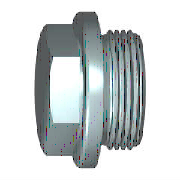
# Autodesk Inventor part: CSN 02 1915.21 - M 20 x 10
Saved by Autodesk Inventor 2016 (Build 200138000, 138)
## iProperties
Created: 2015-02-19
Part Number: CSN 02 1915.21 - M 20 x 10
Material: Сталь, мягкая
Description: Пробка резьбовая с цилиндрической резьбой
Document SubType Name: Modeling
Standard: CSN 02 1915.21
Designer: Лол
Standards Organization: CSN
Language: ru-RU
Size Designation: M 20 x 10
Categories: <MemberInstance><Categories><Category DisplayName="Другие детали" InternalName="5aa15e00-363f-49f2-933f-16f664388e3f" Mnemonic="OTHER"><Category DisplayName="Пробки" InternalName="cac7eb15-d262-4465-a909-3aa76acf7ccc" Mnemonic="PGCLOS"><CategoryParameter DisplayName="Номинальный диаметр" InternalName="0cc7991d-0c39-4ac8-8486-c7d2ae5a3476" Mnemonic="nomdia2"/><CategoryParameter DisplayName="Обозначение серии резьб" InternalName="103883d0-9ece-47bf-a0f3-82d73a20391a" Mnemonic="thrserdsgn2"/><CategoryParameter DisplayName="Шаг резьбы" InternalName="3d473a7f-1ce0-4f16-9b77-af7fe5847f9b" Mnemonic="pitch2"/><CategoryParameter DisplayName="Витков на единицу" InternalName="705c2615-1a74-4f7a-b097-68f368d5139c" Mnemonic="thrperunit2"/><CategoryParameter DisplayName="Класс резьбы" InternalName="af44356c-65bc-4d9d-8b82-abec66cec71c" Mnemonic="thrclss2"/><CategoryParameter DisplayName="Обозначение резьбы" InternalName="d850c9d1-8a6b-401c-92c1-7eca3a245b93" Mnemonic="thrdesign2"/></Category></Category><Category DisplayName="ТипДанных" InternalName="23b78d0f-2648-40c6-8793-ca6db495c9e8" Mnemonic="DATATYPE"><CategoryParameter DisplayName="ОтображаемоеИмя" InternalName="05415f3d-3907-474b-a020-eb9d644f4cf3" Mnemonic="DISPLAYNAME"/><CategoryParameter DisplayName="Стандарт" InternalName="0c0a119c-1e12-4c84-803f-101930972f5e" Mnemonic="STANDARD"/><CategoryParameter DisplayName="Наименование" InternalName="13903e3d-64b1-4950-80da-f627842ea37f" Mnemonic="DESCRIPTION"/><CategoryParameter DisplayName="Обозначение" InternalName="2675968c-4ce5-49e0-a4f5-552d29089031" Mnemonic="DESIGNATION"/><CategoryParameter DisplayName="Строка по умолчанию" InternalName="2af9ec52-faaa-4026-b378-f9fa4afca842" Mnemonic="DEFAULTROW"/><CategoryParameter DisplayName="Имя папки" InternalName="3f06958e-8713-4116-9be7-ed6184ecc97b" Mnemonic="FOLDERNAME"/><CategoryParameter DisplayName="Указатель редакций" InternalName="45a75005-10b1-4dfc-8d6d-dfe629f0b93c" Mnemonic="REVISIONGUID"/><CategoryParameter DisplayName="ИмяФайла" InternalName="8b46a4cc-9585-4fed-90c3-899f57e09a73" Mnemonic="FILENAME"/><CategoryParameter DisplayName="ОргСтанд" InternalName="8f5914e1-4693-403f-8ab5-d37768198c9d" Mnemonic="STDSORG"/><CategoryParameter DisplayName="Версия семейства" InternalName="914462f6-6e19-4b14-ba84-155b9680b1d0" Mnemonic="FAMILYREVISION"/><CategoryParameter DisplayName="Редакция стандарта" InternalName="91d5a463-65c2-4fde-b823-3b7fea5e8e17" Mnemonic="STANDARDREVISION"/><CategoryParameter DisplayName="редакция элемента" InternalName="a65d44b9-392f-4f4f-857b-e4b3d54996fe" Mnemonic="MEMBERREVISION"/><CategoryParameter DisplayName="ФорматКлипа" InternalName="bc51e27b-3422-4e78-93ef-cec197ddf230" Mnemonic="CLIPFORMAT"/><CategoryParameter DisplayName="Изготовитель" InternalName="cd6c7a72-a28a-4e50-99a9-2c7f4e13e5ad" Mnemonic="MANUFACTURER"/><CategoryParameter DisplayName="ВнутреннееИмя" InternalName="cf1d0246-76d9-4b4a-8305-fa0409afb5c1" Mnemonic="INTERNALNAME"/><CategoryParameter DisplayName="Метрическая" InternalName="e2385c5b-1ea4-4823-96a8-8de651266ec3" Mnemonic="ISMETRIC"/><Category DisplayName="Деталь" InternalName="c0e0b642-3bcb-4cc8-9e80-f96d35c4afa4" Mnemonic="PART"><CategoryParameter DisplayName="Номер детали" InternalName="016b6077-bfbe-49bd-92c9-d8d59c39c941" Mnemonic="PARTNUMBER"/><CategoryParameter DisplayName="Инвентарный номер" InternalName="4dba7c1c-e26c-444e-836c-b08b433409a8" Mnemonic="STOCKNUMBER"/><CategoryParameter DisplayName="Ключ материала" InternalName="5c9a8adb-dd2b-4535-b97f-0a94a95fe41f" Mnemonic="MATERIALKEY"/><CategoryParameter DisplayName="Материал" InternalName="818a152a-d3c3-49ca-80ee-df7d91421b8e" Mnemonic="MATERIAL"/></Category></Category><Category DisplayName="СтараяКарта" InternalName="cd87c42b-3e48-431e-b5c0-1cbeb14dfe77" Mnemonic="LEGACYMAP"><CategoryParameter DisplayName="уникальное обозначение элемента DA" InternalName="0918ad47-427f-4fed-ae26-24c81c58f590" Mnemonic="DACOOKIE"/><CategoryParameter DisplayName="Объединить код 11" InternalName="0ee8fb18-e2ed-4f39-96f6-1f4b5f50aa71" Mnemonic="MERGE11"/><CategoryParameter DisplayName="уникальное обозначение элемента CC" InternalName="5193edd4-b2b0-4ab4-9d54-de900eee34e0" Mnemonic="CCCOOKIE"/><CategoryParameter DisplayName="Разделить код" InternalName="72b5c83c-be7f-45c4-ae51-9160ea6deb26" Mnemonic="SPLIT"/><CategoryParameter DisplayName="КодУчастника" InternalName="8e5e0294-fc51-4c8f-b3d7-003dc5ed94f6" Mnemonic="MEMBERID"/><CategoryParameter DisplayName="ИмяКаталога" InternalName="d99d1e27-aa94-4de2-af4c-c348882a6f4f" Mnemonic="CATALOGNAME"/><CategoryParameter DisplayName="НомерСемейства" InternalName="e705e1f4-09cb-413e-91f9-551b4188271e" Mnemonic="FAMILYNUMBER"/></Category></Categories><FamilyTemplate Id="si0169"><FamilyTemplateParameters><FamilyTemplateParameter ObjectType="kUserParameterObject" ValueType="xs:double" Id="1" ObjectReferenceKey="GUL"/><FamilyTemplateParameter ObjectType="kUserParameterObject" ValueType="xs:double" Id="2" ObjectReferenceKey="KOH"/><FamilyTemplateParameter ObjectType="kUserParameterObject" ValueType="xs:double" Id="3" ObjectReferenceKey="NLG"/><FamilyTemplateParameter ObjectType="kUserParameterObject" ValueType="xs:double" Id="4" ObjectReferenceKey="KOD"/><FamilyTemplateParameter ObjectType="kUserParameterObject" ValueType="xs:double" Id="5" ObjectReferenceKey="PHH"/><FamilyTemplateParameter ObjectType="kUserParameterObject" ValueType="xs:double" Id="6" ObjectReferenceKey="GEL"/><FamilyTemplateParameter ObjectType="kUserParameterObject" ValueType="xs:double" Id="7" ObjectReferenceKey="SW"/><FamilyTemplateParameter ObjectType="kUserParameterObject" ValueType="xs:double" Id="8" ObjectReferenceKey="THREADDIA"/><FamilyTemplateParameter ObjectType="kUserParameterObject" ValueType="xs:double" Id="9" ObjectReferenceKey="TOA"/><FamilyTemplateParameter ObjectType="kUserParameterObject" ValueType="xs:double" Id="10" ObjectReferenceKey="RR"/><FamilyTemplateParameter ObjectType="kUserParameterObject" ValueType="xs:double" Id="11" ObjectReferenceKey="TPU"/><FamilyTemplateParameter ObjectType="kUserParameterObject" ValueType="xs:double" Id="12" ObjectReferenceKey="PTC"/><FamilyTemplateParameter ObjectType="kUserParameterObject" ValueType="xs:double" Id="13" ObjectReferenceKey="NND"/><FamilyTemplateParameter ObjectType="kUserParameterObject" ValueType="xs:double" Id="14" ObjectReferenceKey="GAL1"/><FamilyTemplateParameter ObjectType="kUserParameterObject" ValueType="xs:double" Id="15" ObjectReferenceKey="GAL"/><FamilyTemplateParameter ObjectType="kUserParameterObject" ValueType="xs:double" Id="16" ObjectReferenceKey="SD"/><FamilyTemplateParameter ObjectType="kUserParameterObject" ValueType="xs:double" Id="17" ObjectReferenceKey="GD1"/><FamilyTemplateParameter ObjectType="kPropertyObject" ValueType="xs:string" Id="100" ObjectReferenceKey="{32853F0F-3444-11d1-9E93-0060B03C1CA6}" SubObjectId="52"/><FamilyTemplateParameter ObjectType="kPropertyObject" ValueType="xs:string" Id="105" ObjectReferenceKey="{32853F0F-3444-11d1-9E93-0060B03C1CA6}" SubObjectId="5"/><FamilyTemplateParameter ObjectType="kPartComponentDefinitionObject" ValueType="xs:string" Id="110" SubObjectId="Material"/><FamilyTemplateParameter ObjectType="kThreadFeatureObject" ValueType="xs:structure" Id="300" ObjectReferenceKey="100200001000000051040000000000008000000000000000" SubObjectId="ThreadInfo"><FamilyTemplateParameter ObjectType="" ValueType="xs:string" Id="301" SubObjectId="ThreadDesignation"/><FamilyTemplateParameter ObjectType="" ValueType="xs:string" Id="302" SubObjectId="ThreadType"/><FamilyTemplateParameter ObjectType="" ValueType="xs:string" Id="303" SubObjectId="ThreadClass"/></FamilyTemplateParameter></FamilyTemplateParameters></FamilyTemplate><CategoryParameterMap><ParamToTemplateMap><ParamToTemplate CategoryParameter="//CategoryParameter[@InternalName='05415f3d-3907-474b-a020-eb9d644f4cf3']" ConstantValue="CSN 02 1915.21 (Fine Thread)"/><ParamToTemplate CategoryParameter="//CategoryParameter[@InternalName='cf1d0246-76d9-4b4a-8305-fa0409afb5c1']" ConstantValue="b375d23f-38d1-4472-af1b-3d577ff944c2"/><ParamToTemplate CategoryParameter="//CategoryParameter[@InternalName='3f06958e-8713-4116-9be7-ed6184ecc97b']" ConstantValue="CSN 02 1915.21  FT"/><ParamToTemplate CategoryParameter="//CategoryParameter[@InternalName='914462f6-6e19-4b14-ba84-155b9680b1d0']" ConstantValue="10"/><ParamToTemplate CategoryParameter="//CategoryParameter[@InternalName='bc51e27b-3422-4e78-93ef-cec197ddf230']" ConstantValue="CF_INVENTOR.STDPARTS"/><ParamToTemplate CategoryParameter="//CategoryParameter[@InternalName='e2385c5b-1ea4-4823-96a8-8de651266ec3']" ConstantValue="true"/><ParamToTemplate CategoryParameter="//CategoryParameter[@InternalName='13903e3d-64b1-4950-80da-f627842ea37f']" ConstantValue="Screw plug with cylindrical thread"/><ParamToTemplate CategoryParameter="//CategoryParameter[@InternalName='8f5914e1-4693-403f-8ab5-d37768198c9d']" ConstantValue="CSN"/><ParamToTemplate CategoryParameter="//CategoryParameter[@InternalName='0c0a119c-1e12-4c84-803f-101930972f5e']" ConstantValue="CSN 02 1915.21"/><ParamToTemplate CategoryParameter="//CategoryParameter[@InternalName='cd6c7a72-a28a-4e50-99a9-2c7f4e13e5ad']" TemplateParameter="104"/><ParamToTemplate CategoryParameter="//CategoryParameter[@InternalName='91d5a463-65c2-4fde-b823-3b7fea5e8e17']" TemplateParameter="103"/><ParamToTemplate CategoryParameter="//CategoryParameter[@InternalName='45a75005-10b1-4dfc-8d6d-dfe629f0b93c']" ConstantValue="ec25bdad-d347-4146-a37b-df0996dfe8d7"/><ParamToTemplate CategoryParameter="//CategoryParameter[@InternalName='2af9ec52-faaa-4026-b378-f9fa4afca842']" ConstantValue="1"/><ParamToTemplate CategoryParameter="//CategoryParameter[@InternalName='d99d1e27-aa94-4de2-af4c-c348882a6f4f']" ConstantValue="CSN"/><ParamToTemplate CategoryParameter="//CategoryParameter[@InternalName='e705e1f4-09cb-413e-91f9-551b4188271e']" ConstantValue="106"/><ParamToTemplate CategoryParameter="//CategoryParameter[@InternalName='8b46a4cc-9585-4fed-90c3-899f57e09a73']" ConstantValue="CSN 02 1915.21 - M 20 x 10"/><ParamToTemplate CategoryParameter="//CategoryParameter[@InternalName='a65d44b9-392f-4f4f-857b-e4b3d54996fe']" ConstantValue="8b0c0261-c758-4e1b-b85b-8253fe0b580c"/><ParamToTemplate CategoryParameter="//CategoryParameter[@InternalName='af44356c-65bc-4d9d-8b82-abec66cec71c']" ConstantValue="6g"/><ParamToTemplate CategoryParameter="//CategoryParameter[@InternalName='8e5e0294-fc51-4c8f-b3d7-003dc5ed94f6']" ConstantValue="1"/><ParamToTemplate CategoryParameter="//CategoryParameter[@InternalName='2675968c-4ce5-49e0-a4f5-552d29089031']" TemplateParameter="100"/><ParamToTemplate CategoryParameter="//CategoryParameter[@InternalName='818a152a-d3c3-49ca-80ee-df7d91421b8e']" TemplateParameter="110"/><ParamToTemplate CategoryParameter="//CategoryParameter[@InternalName='0cc7991d-0c39-4ac8-8486-c7d2ae5a3476']" TemplateParameter="13"/><ParamToTemplate CategoryParameter="//CategoryParameter[@InternalName='016b6077-bfbe-49bd-92c9-d8d59c39c941']" TemplateParameter="105"/><ParamToTemplate CategoryParameter="//CategoryParameter[@InternalName='3d473a7f-1ce0-4f16-9b77-af7fe5847f9b']" TemplateParameter="12"/><ParamToTemplate CategoryParameter="//CategoryParameter[@InternalName='d850c9d1-8a6b-401c-92c1-7eca3a245b93']" TemplateParameter="301"/><ParamToTemplate CategoryParameter="//CategoryParameter[@InternalName='705c2615-1a74-4f7a-b097-68f368d5139c']" TemplateParameter="11"/></ParamToTemplateMap></CategoryParameterMap></MemberInstance>
Density: 7.85 g/cm^3
Appearance: С умеренной полировкой
IsCustomPart: 0
Author: Лол
Autodesk Inventor part; units mm, degrees
ref_plane "YZ Plane" through (0, 0, 0) normal (1, 0, 0) x (0, 1, 0)
ref_plane "XZ Plane" through (0, 0, 0) normal (0, 1, 0) x (-1, 0, 0)
ref_plane "XY Plane" through (0, 0, 0) normal (0, 0, 1) x (1, 0, 0)
sketch "Эскиз1" plane through (0, 0, 0) normal (0, 0, 1) x (1, 0, 0)
  line L0 (10, 0) -> (10, 10)
  line L1 (10, 10) -> (3, 10)
  line L2 (3, 10) -> (1.8448, 9.1888)
  line L3 (1.1552, 9.1888) -> (0, 10)
  line L4 (0, 10) -> (0, 13)
  line L5 (0, 13) -> (-4, 13)
  line L6 (-4, 13) -> (-4, 10.9697)
  line L7 (-4, 10.9697) -> (-4.8, 10.9697)
  line L8 (-4.8, 10.9697) -> (-4.8, 0)
  line L9 (-4.8, 0) -> (10, 0)
  arc A0 (1.1552, 9.1888) -> (1.8448, 9.1888) centre (1.5, 9.6798) ccw
  line L10 (-7.8876, 0) -> (13.7255, 0) projected
  line L11 (0, -2.6) -> (0, 15.6) projected
  line L12 (2.3733, 9.0798) -> (10.6379, 9.0798) construction
  dimension "d0" = 0.6
  dimension "d1" = 20
  dimension "d2" = 26
  dimension "d3" = 10
  dimension "d4" = 3
  dimension "d5" = 1.5
  dimension "d6" = 21.9393
  dimension "d7" = 4
  dimension "d8" = 0.8
  dimension "d10" = 18.1596
  constraints: 22 end point, 6 parallel, 3 tangent, 2 collinear, 2 perpendicular, 2 point on circle, 1 centre point, 1 point on line, 1 vertical
  measures "d0" radius of A0
  measures "d1" diameter of L1 L9
  measures "d2" diameter of L5 L9
  measures "d3" distance between parallel lines of L0 L4
  measures "d4" distance from line of L1.end L4
  measures "d5" horizontal distance of L1.end A0.centre
  measures "d6" diameter of L7 L9
  measures "d7" distance of L4.end L5.end
  measures "d8" distance of L6.end L7.end
  measures "d10" diameter of L12 L9
revolve "Базовый элемент" add sketch "Эскиз1" angle 360 about axis through (-4.8, 0, 0) along (1, 0, 0)
sketch "Эскиз2" plane through (-4.8, 0, 0) normal (-1, 0, 0) x (0, 0, 1)
  circle A0 centre (0, 0) radius 10.9697 projected
  line L0 (10.9697, 0) -> (5.4848, -9.5)
  line L1 (5.4848, -9.5) -> (-5.4848, -9.5)
  line L2 (-5.4848, -9.5) -> (-10.9697, 0)
  line L3 (-10.9697, 0) -> (-5.4848, 9.5)
  line L4 (-5.4848, 9.5) -> (5.4848, 9.5)
  line L5 (5.4848, 9.5) -> (10.9697, 0)
  constraints: 12 end point, 1 coincident, 1 horizontal, 1 horizontal alignment, 12 other
extrude "С головкой" add sketch "Эскиз2" along normal blind 7 contours L0 L1 L2 L3 L4 L5
fillet "Сопряжение1" radius 1 1 edges at (-4, -13, 0)
sketch "Эскиз3" plane through (0, 0, 0) normal (0, 1, 0) x (-1, 0, 0)
  line L0 (10.75, 10.9697) -> (11.8, 9.151)
  line L1 (11.8, 9.151) -> (11.8, 10.9697)
  line L2 (11.8, 10.9697) -> (10.75, 10.9697)
  line L3 (12.01, 0) -> (10.54, 0) projected
  dimension "d14" = 1.05
  dimension "d15" = 30
  constraints: 6 end point, 1 coincident, 1 perpendicular, 1 vertical
  measures "d14" distance of L1.end L0.start
  measures "d15" angle of L1 L0
revolve "Фаска1" cut sketch "Эскиз3" angle 360 about axis through (-10, 0, 0) along (1, 0, 0)
thread "Резьба1" size "M20x1.5" class "6g" standard "ISO Metric profile" length 10
chamfer "Фаска2" distance 0.9202 distance2 0.9202 1 edges at (10, -10, 0) measured on face at (9.5, -10, 0)
equation "\"d12\" = KOH"
equation "\"d14\" = 0.15 * KOH"
equation "\"d17\" = RR"
equation "\"d20\" = NLG"
equation "\"d18\" = GAL"
equation "\"d19\" = -0.5 * GD1 + 0.5 * NND"
equation "\"d0\" = 0.2 * GAL1"
equation "\"d1\" = NND"
equation "\"d2\" = KOD"
equation "\"d3\" = NLG"
equation "\"d4\" = GAL1"
equation "\"d5\" = 0.5 * GAL1"
equation "\"d6\" = n_D"
equation "\"d7\" = SD"
equation "\"d8\" = PHH"
equation "\"d10\" = GD1"
equation "\"NLG\" = 10"
equation "\"NND\" = 20"
equation "\"SD\" = 4"
equation "\"PHH\" = 0.8"
equation "\"SW\" = 19"
equation "\"GAL1\" = 3"
equation "\"KOH\" = 7"
equation "\"KOD\" = 26"
equation "\"GAL\" = 0.61345 * PTC"
equation "\"RR\" = 1"
equation "\"GD1\" = THREADDIA - 1.2269 * PTC"
equation "\"n_D\" = 1.1547 * SW"
equation "\"GUL\" = 0.61345 * PTC"
equation "\"TOA\" = 30deg"
equation "\"PTC\" = 1.5"
equation "\"THREADDIA\" = 20"
body "Solid1"
